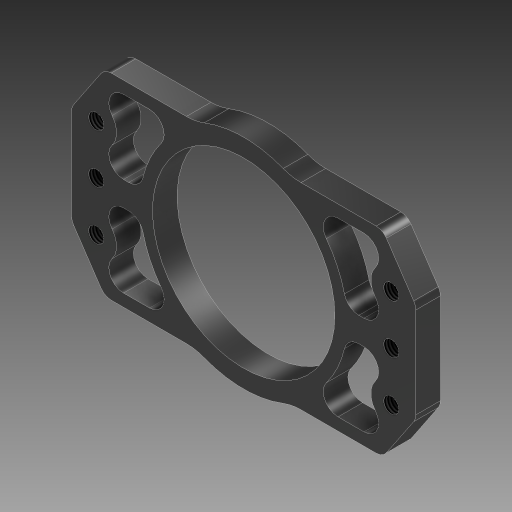
# Autodesk Inventor part: MaxSpline Bearing Block V2
Saved by Autodesk Inventor 2024 (Build 280153000, 153)
## iProperties
Created: 2023-06-08
Part Number: MaxSpline Bearing Block V2
Material: Aluminum 6061
Document SubType Name: Modeling
Designer: Max Boord
Mass: 30.6823 g
Surface Area: 80.6531 cm^2
Volume: 11.3638 cm^3
Density: 2.7 g/cm^3
Appearance: Glossy - Black
Author: Max Boord
Mass: 38.2233 g
Surface Area: 90.3275 cm^2
Volume: 14.1568 cm^3
Mass: 45.745 g
Surface Area: 120.143 cm^2
Volume: 16.9426 cm^3
Autodesk Inventor part; units mm, degrees
ref_plane "YZ Plane" through (0, 0, 0) normal (1, 0, 0) x (0, 1, 0)
ref_plane "XZ Plane" through (0, 0, 0) normal (0, 1, 0) x (-1, 0, 0)
ref_plane "XY Plane" through (0, 0, 0) normal (0, 0, 1) x (1, 0, 0)
sketch "98455A727" plane through (0, 0, 0) normal (0, 0, 1) x (1, 0, 0)
  arc A0 (6.9432, -19.2352) -> (14.6893, -14.3571) centre (-11.4447, 18.5524) ccw
  line L0 (6.9432, -19.2352) -> (8.5729, -23.7501)
  arc A1 (8.5729, -23.7501) -> (-8.5729, -23.7501) centre (0, 0) ccw
  line L1 (-8.5729, -23.7501) -> (-6.9432, -19.2352)
  arc A2 (-14.6893, -14.3571) -> (-6.9432, -19.2352) centre (11.4447, 18.5524) ccw
  arc A3 (-19.2113, -12.7369) -> (-14.6893, -14.3571) centre (-15.9789, -10.8358) ccw
  arc A4 (19.2113, -12.7369) -> (-19.2113, -12.7369) centre (0, -1.4378) ccw
  arc A5 (14.6893, -14.3571) -> (19.2113, -12.7369) centre (15.9789, -10.8358) ccw
  circle A6 centre (11.6445, -18.4904) radius 1.25
  circle A7 centre (-11.6445, -18.4904) radius 1.25
  point P0 (0, 0)
sketch "MaxSpline" plane through (0, 0, 0) normal (0, 0, 1) x (1, 0, 0)
  arc A0 (5.3054, -13.2525) -> (8.8243, -11.2209) centre (0, 0) ccw
  arc A1 (-8.8243, -11.2209) -> (-5.3054, -13.2525) centre (0, 0) ccw
  arc A2 (-14.1297, 2.0316) -> (-14.1297, -2.0316) centre (0, 0) ccw
  arc A3 (-5.3054, 13.2525) -> (-8.8243, 11.2209) centre (0, 0) ccw
  arc A4 (8.8243, 11.2209) -> (5.3054, 13.2525) centre (0, 0) ccw
  arc A5 (-4.7209, 11.79) -> (-2.436, 15.2723) centre (-6.072, 15.1672) ccw
  arc A6 (-2.0329, 15.7443) -> (-2.436, 15.2723) centre (-1.9737, 15.2856) ccw
  arc A7 (2.0329, 15.7443) -> (-2.0329, 15.7443) centre (0, 0) ccw
  arc A8 (2.436, 15.2723) -> (2.0329, 15.7443) centre (1.9737, 15.2856) ccw
  arc A9 (2.436, 15.2723) -> (4.7201, 11.7903) centre (6.072, 15.1672) ccw
  arc A10 (7.8507, 9.9828) -> (4.7201, 11.7903) centre (0, 0) ccw
  arc A11 (7.8507, 9.9828) -> (12.0082, 9.7457) centre (10.0992, 12.8421) ccw
  arc A12 (12.6185, 9.6327) -> (12.0082, 9.7457) centre (12.2509, 9.3521) ccw
  arc A13 (14.6514, 6.1116) -> (12.6185, 9.6327) centre (0, 0) ccw
  arc A14 (14.4442, 5.5265) -> (14.6514, 6.1116) centre (14.2246, 5.9336) ccw
  arc A15 (14.4442, 5.5265) -> (12.5707, 1.8075) centre (16.1712, 2.3251) ccw
  arc A16 (12.5707, -1.8075) -> (12.5707, 1.8075) centre (0, 0) ccw
  arc A17 (12.5707, -1.8075) -> (14.4442, -5.5265) centre (16.1712, -2.3251) ccw
  arc A18 (14.6514, -6.1116) -> (14.4442, -5.5265) centre (14.2246, -5.9336) ccw
  arc A19 (12.6185, -9.6327) -> (14.6514, -6.1116) centre (0, 0) ccw
  arc A20 (12.0082, -9.7457) -> (12.6185, -9.6327) centre (12.2509, -9.3521) ccw
  arc A21 (12.0082, -9.7457) -> (7.8507, -9.9828) centre (10.0992, -12.8421) ccw
  arc A22 (4.7201, -11.7903) -> (7.8507, -9.9828) centre (0, 0) ccw
  arc A23 (4.7201, -11.7903) -> (2.436, -15.2723) centre (6.072, -15.1672) ccw
  arc A24 (2.0329, -15.7443) -> (2.436, -15.2723) centre (1.9737, -15.2856) ccw
  arc A25 (-2.0329, -15.7443) -> (2.0329, -15.7443) centre (0, 0) ccw
  arc A26 (-2.436, -15.2723) -> (-2.0329, -15.7443) centre (-1.9737, -15.2856) ccw
  arc A27 (-2.436, -15.2723) -> (-4.7201, -11.7903) centre (-6.072, -15.1672) ccw
  arc A28 (-7.8507, -9.9828) -> (-4.7201, -11.7903) centre (0, 0) ccw
  arc A29 (-7.8507, -9.9828) -> (-12.0082, -9.7457) centre (-10.0992, -12.8421) ccw
  arc A30 (-12.6185, -9.6327) -> (-12.0082, -9.7457) centre (-12.2509, -9.3521) ccw
  arc A31 (-14.6514, -6.1116) -> (-12.6185, -9.6327) centre (0, 0) ccw
  arc A32 (-14.4442, -5.5265) -> (-14.6514, -6.1116) centre (-14.2246, -5.9336) ccw
  arc A33 (-14.4442, -5.5265) -> (-12.5707, -1.8075) centre (-16.1712, -2.3251) ccw
  arc A34 (-12.5707, 1.8075) -> (-12.5707, -1.8075) centre (0, 0) ccw
  arc A35 (-12.5707, 1.8075) -> (-14.4442, 5.5265) centre (-16.1712, 2.3251) ccw
  arc A36 (-14.6514, 6.1116) -> (-14.4442, 5.5265) centre (-14.2246, 5.9336) ccw
  arc A37 (-12.6185, 9.6327) -> (-14.6514, 6.1116) centre (0, 0) ccw
  arc A38 (-12.0082, 9.7457) -> (-12.6185, 9.6327) centre (-12.2509, 9.3521) ccw
  arc A39 (-12.0082, 9.7457) -> (-7.8507, 9.9828) centre (-10.0992, 12.8421) ccw
  arc A40 (-4.7172, 11.7914) -> (-7.8507, 9.9828) centre (0, 0) ccw
  line L0 (0, 0) -> (0, 22.7025) construction
  line L1 (-1.9737, 15.2856) -> (0, 0) construction
  line L2 (1.9737, 15.2856) -> (0, 0) construction
  line L3 (-10.0992, 12.8421) -> (0, 0) construction
  line L4 (-6.072, 15.1672) -> (0, 0) construction
  arc A41 (2.2346, 17.3063) -> (-2.2346, 17.3063) centre (0, 0) ccw
  arc A42 (16.105, 6.718) -> (13.8704, 10.5884) centre (0, 0) ccw
  arc A43 (13.8704, -10.5884) -> (16.105, -6.718) centre (0, 0) ccw
  arc A44 (-2.2346, -17.3063) -> (2.2346, -17.3063) centre (0, 0) ccw
  arc A45 (-13.8704, 10.5884) -> (-16.105, 6.718) centre (0, 0) ccw
  arc A46 (-16.105, -6.718) -> (-13.8704, -10.5884) centre (0, 0) ccw
  arc A47 (14.1297, -2.0316) -> (14.1297, 2.0316) centre (0, 0) ccw
  dimension "d113" = 360
  dimension "d114" = 2.0375
  dimension "d115" = 2.0625
  dimension "d108" = 14.715
  dimension "d109" = 16.364
  dimension "d110" = 34.9
  dimension "d111" = 28.55
  dimension "d112" = 25.4
  measures "d108" angle of L2 L1
  measures "d109" angle of L3 L4
  measures "d110" diameter of A41
  measures "d111" diameter of A4
  measures "d112" diameter of A10
sketch "Sketch2" plane through (0, 0, 0) normal (0, 0, 1) x (1, 0, 0)
  line L0 (-44.45, 25.4) -> (-44.45, -25.3997)
  circle A0 centre (38.1, 12.7) radius 1.27
  line L1 (44.45, -25.4) -> (-44.45, -25.4)
  line L2 (-44.45, -25.4) -> (-44.45, 25.4)
  line L3 (-44.45, 25.4) -> (44.45, 25.4)
  line L4 (44.45, 25.4) -> (44.45, -25.4)
  line L5 (44.45, -25.4) -> (-44.45, 25.4) construction
  line L6 (-44.45, -25.4) -> (44.45, 25.4) construction
  line L7 (0, 0) -> (0, 25.4) construction
  circle A1 centre (-38.1, -12.7) radius 1.27
  circle A2 centre (-38.1, 12.7) radius 1.27
  circle A3 centre (38.1, -12.7) radius 1.27
  circle A4 centre (0, 0) radius 23.55
  circle A5 centre (0, 0) radius 17.78
  circle A6 centre (0, 0) radius 25 construction
  circle A7 centre (38.1, 12.7) radius 5.2705 construction
  circle A8 centre (-38.1, -12.7) radius 5.2705 construction
  circle A9 centre (-38.1, 12.7) radius 5.2705 construction
  circle A10 centre (38.1, -12.7) radius 5.2705 construction
  line L8 (-44.45, 12.7) -> (-35.9155, 25.4)
  line L9 (44.45, -12.7) -> (35.9155, -25.4)
  line L10 (44.45, 12.7) -> (35.9155, 25.4)
  line L11 (-44.45, -12.7) -> (-35.9155, -25.4)
  circle A11 centre (0, 0) radius 28.175
  circle A12 centre (38.1, 0) radius 1.27
  circle A13 centre (-38.1, 0) radius 1.27
  point P0 (-44.582, -25.3997)
  point P1 (-44.45, 0)
  point P2 (-127, 12.7)
  point P3 (-127, -12.7)
  point P4 (44.45, -12.7)
  point P5 (-44.45, 0)
  dimension "d7" = 2.54
  dimension "d15" = 360
  dimension "d17" = 76.2
  dimension "d18" = 25.4
  dimension "d19" = 47.1
  dimension "d20" = 35.56
  dimension "d21" = 6.35
  dimension "d22" = 50
  dimension "d26" = 360
  dimension "d28" = 10.541
  dimension "d33" = 360
  dimension "d36" = 3.175
  dimension "d37" = 25.4
  dimension "d58" = 50.8
  dimension "d59" = 6.35
  constraints: 22 end point, 14 centre point, 9 symmetric about line, 4 midpoint, 3 coincident, 2 horizontal alignment, 2 parallel, 2 point on line, 1 equal radius, 1 horizontal, 1 perpendicular, 1 tangent, 1 vertical alignment, 24 other
  measures "d7" diameter of A0
  measures "d17" distance of A0.centre A2.centre
  measures "d18" distance of A1.centre A2.centre
  measures "d19" diameter of A4
  measures "d20" diameter of A5
  measures "d22" diameter of A6
  measures "d28" diameter of A7
  measures "d36" radial gap between concentric circles of A6 A11
  measures "d37" distance of L11.start L8.start
  measures "d58" distance between parallel lines of L3 L1
  measures "d59" distance from line of A2.centre L2
extrude "Extrusion3" add sketch "Sketch2" along normal mid plane 6.35 contours L8 L3 A11 L1 L11 L0 | A11 L3 | L3 A11 L1 | L3 L10 L4 L9 L1 A11 | L1 A11
sketch "Sketch3" plane through (0, 0, 3.175) normal (0, 0, 1) x (1, 0, 0)
  point P0 (0, 0)
fillet "Fillet2" radius 3.175 8 edges at (-35.9155, -25.4, 0) (-44.45, -12.7, 0) (-44.45, 12.7, 0) (-35.9155, 25.4, 0) (35.9155, 25.4, 0) (44.45, 12.7, 0) (44.45, -12.7, 0) (35.9155, -25.4, 0)
fillet "Fillet2" radius 12.7 4 edges at (-12.1931, -25.4, 0) (12.1931, -25.4, 0) (12.1931, 25.4, 0) (-12.1931, 25.4, 0)
sketch "Sketch6" plane through (0, 0, 3.175) normal (0, 0, 1) x (1, 0, 0)
  arc A0 (34.2239, -25.4) -> (36.8591, -23.9959) centre (34.2239, -22.225) ccw projected
  line L0 (36.8591, -23.9959) -> (43.9102, -13.5032) projected
  arc A1 (43.9102, -13.5032) -> (44.45, -11.7323) centre (41.275, -11.7323) ccw projected
  line L1 (44.45, -11.7323) -> (44.45, 11.7323) projected
  arc A2 (44.45, 11.7323) -> (43.9102, 13.5032) centre (41.275, 11.7323) ccw projected
  line L2 (43.9102, 13.5032) -> (36.8591, 23.9959) projected
  arc A3 (36.8591, 23.9959) -> (34.2239, 25.4) centre (34.2239, 22.225) ccw projected
  line L3 (34.2239, 25.4) -> (14.8039, 25.4) projected
  arc A4 (10.2043, 26.2622) -> (14.8039, 25.4) centre (14.8039, 38.1) ccw projected
  arc A5 (10.2043, 26.2622) -> (-10.2043, 26.2622) centre (0, 0) ccw projected
  arc A6 (-14.8039, 25.4) -> (-10.2043, 26.2622) centre (-14.8039, 38.1) ccw projected
  line L4 (-14.8039, 25.4) -> (-34.2239, 25.4) projected
  arc A7 (-34.2239, 25.4) -> (-36.8591, 23.9959) centre (-34.2239, 22.225) ccw projected
  line L5 (-36.8591, 23.9959) -> (-43.9102, 13.5032) projected
  arc A8 (-43.9102, 13.5032) -> (-44.45, 11.7323) centre (-41.275, 11.7323) ccw projected
  line L6 (-44.45, 11.7323) -> (-44.45, -11.7323) projected
  arc A9 (-44.45, -11.7323) -> (-43.9102, -13.5032) centre (-41.275, -11.7323) ccw projected
  line L7 (-43.9102, -13.5032) -> (-36.8591, -23.9959) projected
  arc A10 (-36.8591, -23.9959) -> (-34.2239, -25.4) centre (-34.2239, -22.225) ccw projected
  line L8 (-34.2239, -25.4) -> (-14.8039, -25.4) projected
  arc A11 (-10.2043, -26.2622) -> (-14.8039, -25.4) centre (-14.8039, -38.1) ccw projected
  arc A12 (-10.2043, -26.2622) -> (10.2043, -26.2622) centre (0, 0) ccw projected
  arc A13 (14.8039, -25.4) -> (10.2043, -26.2622) centre (14.8039, -38.1) ccw projected
  line L9 (14.8039, -25.4) -> (34.2239, -25.4) projected
  circle A14 centre (0, 0) radius 23.55 projected
  circle A15 centre (38.1, 12.7) radius 1.27 projected
  circle A16 centre (38.1, -12.7) radius 1.27 projected
  circle A17 centre (38.1, 0) radius 1.27 projected
  circle A18 centre (-38.1, -12.7) radius 1.27 projected
  circle A19 centre (-38.1, 12.7) radius 1.27 projected
  circle A20 centre (-38.1, 0) radius 1.27 projected
  circle A21 centre (0, 0) radius 26.725
  line L10 (34.2239, -22.225) -> (41.275, -11.7323)
  line L11 (41.275, -11.7323) -> (41.275, 11.7323)
  line L12 (41.275, 11.7323) -> (34.2239, 22.225)
  line L13 (34.2239, 22.225) -> (14.8039, 22.225)
  arc A22 (9.0544, 23.3028) -> (14.8039, 22.225) centre (14.8039, 38.1) ccw
  arc A23 (9.0544, 23.3028) -> (-9.0544, 23.3028) centre (0, 0) ccw
  arc A24 (-14.8039, 22.225) -> (-9.0544, 23.3028) centre (-14.8039, 38.1) ccw
  line L14 (-14.8039, 22.225) -> (-34.2239, 22.225)
  line L15 (-34.2239, 22.225) -> (-41.275, 11.7323)
  line L16 (-41.275, 11.7323) -> (-41.275, -11.7323)
  line L17 (-41.275, -11.7323) -> (-34.2239, -22.225)
  line L18 (-34.2239, -22.225) -> (-14.8039, -22.225)
  arc A25 (-9.0544, -23.3028) -> (-14.8039, -22.225) centre (-14.8039, -38.1) ccw
  arc A26 (-9.0544, -23.3028) -> (9.0544, -23.3028) centre (0, 0) ccw
  arc A27 (14.8039, -22.225) -> (9.0544, -23.3028) centre (14.8039, -38.1) ccw
  line L19 (14.8039, -22.225) -> (34.2239, -22.225)
  circle A28 centre (38.1, -12.7) radius 5.2705
  circle A29 centre (38.1, 0) radius 5.2705
  circle A30 centre (38.1, 12.7) radius 5.2705
  line L20 (38.1, 0) -> (0, 0) construction
  line L21 (38.1, 3.175) -> (0, 3.175)
  line L22 (0, -3.175) -> (38.1, -3.175)
  arc A31 (38.1, -3.175) -> (38.1, 3.175) centre (38.1, 0) ccw
  arc A32 (0, 3.175) -> (0, -3.175) centre (0, 0) ccw
  line L23 (38.1, -12.7) -> (38.1, 12.7) construction
  line L24 (40.4813, -12.7) -> (40.4813, 12.7)
  line L25 (35.7188, 12.7) -> (35.7188, -12.7)
  arc A33 (35.7188, -12.7) -> (40.4813, -12.7) centre (38.1, -12.7) ccw
  arc A34 (40.4813, 12.7) -> (35.7188, 12.7) centre (38.1, 12.7) ccw
  point P0 (19.05, 0)
  point P1 (38.1, 0)
  point P2 (35.7188, 4.7019)
  point P3 (35.7188, 7.9981)
  point P4 (37.1419, 17.8827)
  point P5 (14.8417, 22.225)
  point P6 (26.5357, 3.175)
  point P7 (33.8932, 3.175)
  point P8 (35.7188, -7.9981)
  point P9 (35.7188, -4.7019)
  point P10 (33.8932, -3.175)
  point P11 (26.5357, -3.175)
  point P12 (14.8417, -22.225)
  point P13 (37.1419, -17.8827)
  dimension "d62" = 3.175
  dimension "d63" = 3.175
  dimension "d64" = 10.541
  dimension "d65" = 6.35
  dimension "d66" = 4.7625
  constraints: 36 end point, 20 point on circle, 14 centre point, 8 tangent, 2 equal radius, 2 midpoint, 2 parallel, 1 horizontal, 1 perpendicular, 15 other
  measures "d62" radial gap between concentric circles of A14 A21
  measures "d63" distance between parallel lines of L9 L19
  measures "d64" diameter of A28
  measures "d65" diameter of A32
  measures "d66" diameter of A34
extrude "Extrusion5" cut sketch "Sketch6" against normal through all contours L10 L19 A21 L22 A29 L25 A28 | L21 A21 L13 L12 A30 L25 A29
fillet "Fillet3" radius 3.81 14 edges at (33.8932, 3.175, 0) (35.7188, 4.7019, 0) (35.7188, 7.9981, 0) (37.1419, 17.8827, 0) (34.2239, 22.225, 0) (14.8417, 22.225, 0) (26.5357, 3.175, 0) (37.1419, -17.8827, 0) (35.7188, -7.9981, 0) (35.7188, -4.7019, 0) (33.8932, -3.175, 0) (26.5357, -3.175, 0) (14.8417, -22.225, 0) (34.2239, -22.225, 0)
mirror "Mirror1" about plane through (0, 0, 0) normal (1, 0, 0) of "Fillet3", "Extrusion5"
sketch "Sketch7" plane through (0, 0, 0) normal (0, 1, 0) x (-1, 0, 0)
  line L0 (21.3614, -3.786) -> (21.3614, 2.325)
  line L1 (21.3614, 2.325) -> (27.7114, 2.325)
  line L2 (27.7114, 2.325) -> (27.7114, 3.214)
  line L3 (5.1562, 3.214) -> (5.1562, -3.786)
  line L4 (0, 0) -> (0, 6.5668)
  line L5 (7.5184, 3.214) -> (7.5184, 2.833)
  line L6 (7.5184, 2.833) -> (18.9992, 2.833)
  line L7 (18.9992, 2.833) -> (18.9992, 3.214)
  line L8 (5.1562, -0.286) -> (21.3614, -0.286) construction
  line L9 (7.5184, -3.786) -> (7.5184, -3.405)
  line L10 (7.5184, -3.405) -> (18.9992, -3.405)
  line L11 (18.9992, -3.405) -> (18.9992, -3.786)
  line L12 (27.7114, 3.214) -> (7.5184, 3.214)
  line L13 (18.9992, 3.214) -> (5.1562, 3.214)
  line L14 (5.1562, -3.786) -> (18.9992, -3.786)
  line L15 (7.5184, -3.786) -> (21.3614, -3.786)
  line L16 (0, 3.175) -> (-3.0494, 3.175) construction
  line L17 (0, 0) -> (-3.6555, 0)
  line L18 (0, -3.175) -> (-3.0494, -3.175) construction
  point P0 (5.1562, 4.675)
  point P1 (13.2588, -3.405)
  point P2 (13.2588, -0.286)
  point P3 (7.5184, -3.786)
  point P4 (18.9992, 3.214)
  point P5 (7.5184, 3.214)
  point P6 (18.9992, -3.786)
  point P7 (18.9992, -3.786)
  point P8 (7.5184, 3.214)
  dimension "d72" = 10.3124
  dimension "d73" = 42.7228
  dimension "d74" = 55.4228
  dimension "d84" = 37.9984
  dimension "d85" = 0.889
  dimension "d87" = 0.381
  dimension "d88" = 7
  dimension "d90" = 6.35
  dimension "d91" = 5.5
  constraints: 38 end point, 8 perpendicular, 6 symmetric about line, 5 horizontal, 3 midpoint, 3 point on line, 2 parallel, 1 collinear, 1 vertical, 1 vertical alignment
  measures "d72" diameter of L3 L4
  measures "d73" diameter of L0 L4
  measures "d74" diameter of L2 L4
  measures "d84" diameter of L7 L4
  measures "d85" distance between parallel lines of L12 L1
  measures "d87" distance between parallel lines of L6 L13
  measures "d88" distance of L3.start L3.end
  measures "d90" distance between parallel lines of L18 L16
  measures "d91" distance between parallel lines of L1 L18
revolve "Revolution1" [suppressed]
delete_face "Delete Face1" [suppressed]
ref_plane "Work Plane3" through (0, 0, 3.2258) normal (0, 0, 1) x (1, 0, 0)
sketch "Sketch8" plane through (0, 0, 3.2258) normal (0, 0, 1) x (1, 0, 0)
  circle A0 centre (0, 0) radius 24.75
  dimension "d92" = 49.5
  constraints: 1 centre point, 1 coincident
  measures "d92" diameter of A0
extrude "Extrusion6" [suppressed]
sketch "Sketch9" plane through (0, 0, -3.175) normal (0, 0, -1) x (-1, 0, 0)
  circle A0 centre (0, 0) radius 23.55 projected
  circle A1 centre (0, 0) radius 19.0119
  dimension "d95" = 38.0238
  constraints: 1 centre point
  measures "d95" diameter of A1
extrude "Extrusion7" [suppressed]
sketch "Sketch10" plane through (0, 0, 3.175) normal (0, 0, 1) x (1, 0, 0)
  arc A0 (6.9432, -19.2352) -> (14.6893, -14.3571) centre (-11.4447, 18.5524) ccw
  line L0 (6.9432, -19.2352) -> (8.5729, -23.7501)
  arc A1 (8.5729, -23.7501) -> (-8.5729, -23.7501) centre (0, 0) ccw
  line L1 (-8.5729, -23.7501) -> (-6.9432, -19.2352)
  arc A2 (-14.6893, -14.3571) -> (-6.9432, -19.2352) centre (11.4447, 18.5524) ccw
  arc A3 (-19.2113, -12.7369) -> (-14.6893, -14.3571) centre (-15.9789, -10.8358) ccw
  arc A4 (19.2113, -12.7369) -> (-19.2113, -12.7369) centre (0, -1.4378) ccw
  arc A5 (14.6893, -14.3571) -> (19.2113, -12.7369) centre (15.9789, -10.8358) ccw
  circle A6 centre (11.6445, -18.4904) radius 1.25
  circle A7 centre (-11.6445, -18.4904) radius 1.25
  point P0 (0, 0)
  constraints: 1 other
extrude "Extrusion8" [suppressed]
sketch "Sketch11" plane through (0, 0, 3.175) normal (0, 0, 1) x (1, 0, 0)
  circle A0 centre (-38.1, 12.7) radius 1.27 projected
  circle A1 centre (-38.1, 0) radius 1.27 projected
  circle A2 centre (-38.1, -12.7) radius 1.27 projected
  circle A3 centre (38.1, 12.7) radius 1.27 projected
  circle A4 centre (38.1, 0) radius 1.27 projected
  circle A5 centre (38.1, -12.7) radius 1.27 projected
  point P0 (0, 0)
  constraints: 6 coincident
hole "Hole1" at (-38.1, 12.7, 3.175) at (-38.1, 0, 3.175) at (-38.1, -12.7, 3.175) at (38.1, 12.7, 3.175) at (38.1, 0, 3.175) at (38.1, -12.7, 3.175) direction (0, 0, -1) diameter 3.9624 end through all thread size "10-32 UNF" class "2B" standard "ANSI Unified Screw Threads"
sketch "Sketch12" plane through (0, 0, 3.175) normal (0, 0, 1) x (1, 0, 0)
  circle A0 centre (0, 0) radius 23.55 projected
  arc A1 (10.5884, 13.8704) -> (6.718, 16.105) centre (0, 0) ccw
  arc A2 (6.718, 16.105) -> (4.1403, 15.1919) centre (5.9336, 14.2246) ccw
  arc A3 (2.0316, 14.1297) -> (4.1403, 15.1919) centre (2.3251, 16.1712) ccw
  arc A4 (2.0316, 14.1297) -> (-2.0316, 14.1297) centre (0, 0) ccw
  arc A5 (-4.1403, 15.1919) -> (-2.0316, 14.1297) centre (-2.3251, 16.1712) ccw
  arc A6 (-4.1403, 15.1919) -> (-6.718, 16.105) centre (-5.9336, 14.2246) ccw
  arc A7 (-6.718, 16.105) -> (-10.5884, 13.8704) centre (0, 0) ccw
  arc A8 (-10.5884, 13.8704) -> (-11.0864, 11.1816) centre (-9.3521, 12.2509) ccw
  arc A9 (-11.2209, 8.8243) -> (-11.0864, 11.1816) centre (-12.8421, 10.0992) ccw
  arc A10 (-11.2209, 8.8243) -> (-13.2525, 5.3054) centre (0, 0) ccw
  arc A11 (-15.2268, 4.0103) -> (-13.2525, 5.3054) centre (-15.1672, 6.072) ccw
  arc A12 (-15.2268, 4.0103) -> (-17.3063, 2.2346) centre (-15.2856, 1.9737) ccw
  arc A13 (-17.3063, 2.2346) -> (-17.3063, -2.2346) centre (0, 0) ccw
  arc A14 (-17.3063, -2.2346) -> (-15.2268, -4.0103) centre (-15.2856, -1.9737) ccw
  arc A15 (-13.2525, -5.3054) -> (-15.2268, -4.0103) centre (-15.1672, -6.072) ccw
  arc A16 (-13.2525, -5.3054) -> (-11.2209, -8.8243) centre (0, 0) ccw
  arc A17 (-11.0864, -11.1816) -> (-11.2209, -8.8243) centre (-12.8421, -10.0992) ccw
  arc A18 (-11.0864, -11.1816) -> (-10.5884, -13.8704) centre (-9.3521, -12.2509) ccw
  arc A19 (-10.5884, -13.8704) -> (-6.718, -16.105) centre (0, 0) ccw
  arc A20 (-6.718, -16.105) -> (-4.1403, -15.1919) centre (-5.9336, -14.2246) ccw
  arc A21 (-2.0316, -14.1297) -> (-4.1403, -15.1919) centre (-2.3251, -16.1712) ccw
  arc A22 (-2.0316, -14.1297) -> (2.0316, -14.1297) centre (0, 0) ccw
  arc A23 (4.1403, -15.1919) -> (2.0316, -14.1297) centre (2.3251, -16.1712) ccw
  arc A24 (4.1403, -15.1919) -> (6.718, -16.105) centre (5.9336, -14.2246) ccw
  arc A25 (6.718, -16.105) -> (10.5884, -13.8704) centre (0, 0) ccw
  arc A26 (10.5884, -13.8704) -> (11.0864, -11.1816) centre (9.3521, -12.2509) ccw
  arc A27 (11.2209, -8.8243) -> (11.0864, -11.1816) centre (12.8421, -10.0992) ccw
  arc A28 (11.2209, -8.8243) -> (13.2525, -5.3054) centre (0, 0) ccw
  arc A29 (15.2268, -4.0103) -> (13.2525, -5.3054) centre (15.1672, -6.072) ccw
  arc A30 (15.2268, -4.0103) -> (17.3063, -2.2346) centre (15.2856, -1.9737) ccw
  arc A31 (17.3063, -2.2346) -> (17.3063, 2.2346) centre (0, 0) ccw
  arc A32 (17.3063, 2.2346) -> (15.2268, 4.0103) centre (15.2856, 1.9737) ccw
  arc A33 (13.2525, 5.3054) -> (15.2268, 4.0103) centre (15.1672, 6.072) ccw
  arc A34 (13.2525, 5.3054) -> (11.2209, 8.8243) centre (0, 0) ccw
  arc A35 (11.0864, 11.1816) -> (11.2209, 8.8243) centre (12.8421, 10.0992) ccw
  arc A36 (11.0864, 11.1816) -> (10.5884, 13.8704) centre (9.3521, 12.2509) ccw
  arc A37 (6.1116, 14.6514) -> (5.5265, 14.4442) centre (5.9336, 14.2246) ccw
  arc A38 (9.6327, 12.6185) -> (6.1116, 14.6514) centre (0, 0) ccw
  arc A39 (9.7457, 12.0082) -> (9.6327, 12.6185) centre (9.3521, 12.2509) ccw
  arc A40 (9.7457, 12.0082) -> (9.9828, 7.8507) centre (12.8421, 10.0992) ccw
  arc A41 (11.7903, 4.7201) -> (9.9828, 7.8507) centre (0, 0) ccw
  arc A42 (11.7903, 4.7201) -> (15.2723, 2.436) centre (15.1672, 6.072) ccw
  arc A43 (15.7443, 2.0329) -> (15.2723, 2.436) centre (15.2856, 1.9737) ccw
  arc A44 (15.7443, -2.0329) -> (15.7443, 2.0329) centre (0, 0) ccw
  arc A45 (15.2723, -2.436) -> (15.7443, -2.0329) centre (15.2856, -1.9737) ccw
  arc A46 (15.2723, -2.436) -> (11.7903, -4.7201) centre (15.1672, -6.072) ccw
  arc A47 (9.9828, -7.8507) -> (11.7903, -4.7201) centre (0, 0) ccw
  arc A48 (9.9828, -7.8507) -> (9.7457, -12.0082) centre (12.8421, -10.0992) ccw
  arc A49 (9.6327, -12.6185) -> (9.7457, -12.0082) centre (9.3521, -12.2509) ccw
  arc A50 (6.1116, -14.6514) -> (9.6327, -12.6185) centre (0, 0) ccw
  arc A51 (5.5265, -14.4442) -> (6.1116, -14.6514) centre (5.9336, -14.2246) ccw
  arc A52 (5.5265, -14.4442) -> (1.8075, -12.5707) centre (2.3251, -16.1712) ccw
  arc A53 (-1.8075, -12.5707) -> (1.8075, -12.5707) centre (0, 0) ccw
  arc A54 (-1.8075, -12.5707) -> (-5.5265, -14.4442) centre (-2.3251, -16.1712) ccw
  arc A55 (-6.1116, -14.6514) -> (-5.5265, -14.4442) centre (-5.9336, -14.2246) ccw
  arc A56 (-9.6327, -12.6185) -> (-6.1116, -14.6514) centre (0, 0) ccw
  arc A57 (-9.7457, -12.0082) -> (-9.6327, -12.6185) centre (-9.3521, -12.2509) ccw
  arc A58 (-9.7457, -12.0082) -> (-9.9828, -7.8507) centre (-12.8421, -10.0992) ccw
  arc A59 (-11.7903, -4.7201) -> (-9.9828, -7.8507) centre (0, 0) ccw
  arc A60 (-11.7903, -4.7201) -> (-15.2723, -2.436) centre (-15.1672, -6.072) ccw
  arc A61 (-15.7443, -2.0329) -> (-15.2723, -2.436) centre (-15.2856, -1.9737) ccw
  arc A62 (-15.7443, 2.0329) -> (-15.7443, -2.0329) centre (0, 0) ccw
  arc A63 (-15.2723, 2.436) -> (-15.7443, 2.0329) centre (-15.2856, 1.9737) ccw
  arc A64 (-15.2723, 2.436) -> (-11.7903, 4.7201) centre (-15.1672, 6.072) ccw
  arc A65 (-9.9828, 7.8507) -> (-11.7903, 4.7201) centre (0, 0) ccw
  arc A66 (-9.9828, 7.8507) -> (-9.7457, 12.0082) centre (-12.8421, 10.0992) ccw
  arc A67 (-9.6327, 12.6185) -> (-9.7457, 12.0082) centre (-9.3521, 12.2509) ccw
  arc A68 (-6.1116, 14.6514) -> (-9.6327, 12.6185) centre (0, 0) ccw
  arc A69 (-5.5265, 14.4442) -> (-6.1116, 14.6514) centre (-5.9336, 14.2246) ccw
  arc A70 (-5.5265, 14.4442) -> (-1.8075, 12.5707) centre (-2.3251, 16.1712) ccw
  arc A71 (1.8066, 12.5708) -> (-1.8075, 12.5707) centre (0, 0) ccw
  arc A72 (1.8066, 12.5708) -> (5.5265, 14.4442) centre (2.3251, 16.1712) ccw
  constraints: 1 other
extrude "Extrusion9" [suppressed]
thicken "Thicken1" [suppressed]
delete_face "Delete Face2" [suppressed]
sketch "Sketch13" plane through (-34.2239, -25.4, 3.175) normal (0, 0, 1) x (1, 0, 0)
  line L0 (58.5811, 47.625) -> (65.2674, 47.625) projected
  arc A0 (68.2281, 41.4171) -> (65.2674, 47.625) centre (65.2674, 43.815) ccw projected
  arc A1 (68.2281, 41.4171) -> (68.2281, 34.7829) centre (72.3239, 38.1) ccw projected
  arc A2 (65.2674, 28.575) -> (68.2281, 34.7829) centre (65.2674, 32.385) ccw projected
  line L1 (65.2674, 28.575) -> (63.9492, 28.575) projected
  arc A3 (60.2402, 31.5134) -> (63.9492, 28.575) centre (63.9492, 32.385) ccw projected
  arc A4 (60.2402, 31.5134) -> (55.5419, 41.5173) centre (34.2239, 25.4) ccw projected
  arc A5 (58.5811, 47.625) -> (55.5419, 41.5173) centre (58.5811, 43.815) ccw projected
  line L2 (0, 0) -> (19.42, 0) projected
  arc A6 (68.4477, 0) -> (71.083, 1.4041) centre (68.4477, 3.175) ccw projected
  line L3 (71.083, 1.4041) -> (78.1341, 11.8968) projected
  arc A7 (78.1341, 11.8968) -> (78.6739, 13.6677) centre (75.4989, 13.6677) ccw projected
  line L4 (78.6739, 13.6677) -> (78.6739, 37.1323) projected
  arc A8 (78.6739, 37.1323) -> (78.1341, 38.9032) centre (75.4989, 37.1323) ccw projected
  line L5 (78.1341, 38.9032) -> (71.083, 49.3959) projected
  arc A9 (71.083, 49.3959) -> (68.4477, 50.8) centre (68.4477, 47.625) ccw projected
  line L6 (68.4477, 50.8) -> (49.0278, 50.8) projected
  arc A10 (0, 50.8) -> (-2.6352, 49.3959) centre (0, 47.625) ccw projected
  line L7 (-2.6352, 49.3959) -> (-9.6864, 38.9032) projected
  arc A11 (-9.6864, 38.9032) -> (-10.2261, 37.1323) centre (-7.0511, 37.1323) ccw projected
  line L8 (-10.2261, 37.1323) -> (-10.2261, 13.6677) projected
  arc A12 (-10.2261, 13.6677) -> (-9.6864, 11.8968) centre (-7.0511, 13.6677) ccw projected
  line L9 (-9.6864, 11.8968) -> (-2.6352, 1.4041) projected
  arc A13 (-2.6352, 1.4041) -> (0, 0) centre (0, 3.175) ccw projected
  circle A14 centre (72.3239, 12.7) radius 1.9812 projected
  circle A15 centre (72.3239, 25.4) radius 1.9812 projected
  circle A16 centre (72.3239, 38.1) radius 1.9812 projected
  circle A17 centre (-3.8761, 12.7) radius 1.9812 projected
  circle A18 centre (-3.8761, 25.4) radius 1.9812 projected
  circle A19 centre (-3.8761, 38.1) radius 1.9812 projected
  line L10 (3.1804, 22.225) -> (4.4985, 22.225) projected
  arc A20 (8.2075, 19.2866) -> (4.4985, 22.225) centre (4.4985, 18.415) ccw projected
  arc A21 (8.2075, 19.2866) -> (12.9058, 9.2827) centre (34.2239, 25.4) ccw projected
  arc A22 (9.8666, 3.175) -> (12.9058, 9.2827) centre (9.8666, 6.985) ccw projected
  line L11 (9.8666, 3.175) -> (3.1804, 3.175) projected
  arc A23 (0.2196, 9.3829) -> (3.1804, 3.175) centre (3.1804, 6.985) ccw projected
  arc A24 (0.2196, 9.3829) -> (0.2196, 16.0171) centre (-3.8761, 12.7) ccw projected
  arc A25 (3.1804, 22.225) -> (0.2196, 16.0171) centre (3.1804, 18.415) ccw projected
  line L12 (3.1804, 47.625) -> (9.8666, 47.625) projected
  arc A26 (12.9058, 41.5173) -> (9.8666, 47.625) centre (9.8666, 43.815) ccw projected
  arc A27 (12.9058, 41.5173) -> (8.2075, 31.5134) centre (34.2239, 25.4) ccw projected
  arc A28 (4.4985, 28.575) -> (8.2075, 31.5134) centre (4.4985, 32.385) ccw projected
  line L13 (4.4985, 28.575) -> (3.1804, 28.575) projected
  arc A29 (0.2196, 34.7829) -> (3.1804, 28.575) centre (3.1804, 32.385) ccw projected
  arc A30 (0.2196, 34.7829) -> (0.2196, 41.4171) centre (-3.8761, 38.1) ccw projected
  arc A31 (3.1804, 47.625) -> (0.2196, 41.4171) centre (3.1804, 43.815) ccw projected
  arc A32 (68.2281, 16.0171) -> (68.2281, 9.3829) centre (72.3239, 12.7) ccw projected
  arc A33 (65.2674, 3.175) -> (68.2281, 9.3829) centre (65.2674, 6.985) ccw projected
  line L14 (65.2674, 3.175) -> (58.5811, 3.175) projected
  arc A34 (55.5419, 9.2827) -> (58.5811, 3.175) centre (58.5811, 6.985) ccw projected
  arc A35 (55.5419, 9.2827) -> (60.2402, 19.2866) centre (34.2239, 25.4) ccw projected
  arc A36 (63.9492, 22.225) -> (60.2402, 19.2866) centre (63.9492, 18.415) ccw projected
  line L15 (63.9492, 22.225) -> (65.2674, 22.225) projected
  arc A37 (68.2281, 16.0171) -> (65.2674, 22.225) centre (65.2674, 18.415) ccw projected
  arc A38 (50.3039, 47.625) -> (47.7979, 40.9451) centre (50.3039, 43.815) ccw
  line L16 (50.3039, 47.625) -> (58.5811, 47.625)
  arc A39 (58.5811, 47.625) -> (55.5419, 41.5173) centre (58.5811, 43.815) ccw projected
  line L17 (63.9492, 28.575) -> (57.6523, 28.575)
  arc A40 (54.0011, 31.2964) -> (57.6523, 28.575) centre (57.6523, 32.385) ccw
  arc A41 (60.2402, 31.5134) -> (63.9492, 28.575) centre (63.9492, 32.385) ccw projected
  arc A42 (54.0011, 31.2964) -> (47.7979, 40.9451) centre (34.2239, 25.4) ccw
  arc A43 (44.8729, 39.3499) -> (40.9803, 41.5973) centre (34.2239, 25.4) ccw projected
  line L18 (34.2239, 25.4) -> (34.2239, 31.4123)
  line L19 (34.2239, 25.4) -> (40.9803, 25.4)
  arc A44 (20.6498, 40.9451) -> (18.1438, 47.625) centre (18.1438, 43.815) ccw
  line L20 (18.1438, 47.625) -> (9.8666, 47.625)
  line L21 (4.4985, 28.575) -> (10.7955, 28.575)
  arc A45 (10.7955, 28.575) -> (14.4466, 31.2964) centre (10.7955, 32.385) ccw
  arc A46 (20.6498, 40.9451) -> (14.4466, 31.2964) centre (34.2239, 25.4) ccw
  arc A47 (47.7979, 9.8549) -> (50.3039, 3.175) centre (50.3039, 6.985) ccw
  line L22 (50.3039, 3.175) -> (58.5811, 3.175)
  line L23 (63.9492, 22.225) -> (57.6523, 22.225)
  arc A48 (57.6523, 22.225) -> (54.0011, 19.5036) centre (57.6523, 18.415) ccw
  arc A49 (47.7979, 9.8549) -> (54.0011, 19.5036) centre (34.2239, 25.4) ccw
  arc A50 (18.1438, 3.175) -> (20.6498, 9.8549) centre (18.1438, 6.985) ccw
  arc A51 (14.4466, 19.5036) -> (20.6498, 9.8549) centre (34.2239, 25.4) ccw
  arc A52 (14.4466, 19.5036) -> (10.7955, 22.225) centre (10.7955, 18.415) ccw
  line L24 (4.4985, 22.225) -> (10.7955, 22.225)
  line L25 (18.1438, 3.175) -> (9.8666, 3.175)
  arc A53 (44.4281, 51.6622) -> (49.0278, 50.8) centre (49.0278, 63.5) ccw projected
  arc A54 (44.4281, 51.6622) -> (24.0196, 51.6622) centre (34.2239, 25.4) ccw projected
  arc A55 (19.42, 50.8) -> (24.0196, 51.6622) centre (19.42, 63.5) ccw projected
  line L26 (19.42, 50.8) -> (0, 50.8) projected
  arc A56 (24.0196, -0.8622) -> (19.42, 0) centre (19.42, -12.7) ccw projected
  arc A57 (24.0196, -0.8622) -> (44.4281, -0.8622) centre (34.2239, 25.4) ccw projected
  arc A58 (49.0278, 0) -> (44.4281, -0.8622) centre (49.0278, -12.7) ccw projected
  line L27 (49.0278, 0) -> (68.4477, 0) projected
  point P0 (9.8666, 3.175)
  point P1 (4.4999, 22.225)
  point P2 (4.4985, 28.575)
  dimension "d130" = 41.275
  constraints: 24 point on circle, 22 symmetric about line, 20 end point, 12 centre point, 5 tangent, 2 equal radius, 2 horizontal, 1 concentric, 1 vertical, 9 other
  measures "d130" diameter of A42
extrude "Extrusion10" [suppressed]
sketch "Block3" plane through (0, 0, 0) normal (0, 0, 1) x (1, 0, 0)
  arc A0 (2.2346, 17.3063) -> (-2.2346, 17.3063) centre (0, 0) ccw
  arc A1 (-2.2346, 17.3063) -> (-4.0103, 15.2268) centre (-1.9737, 15.2856) ccw
  arc A2 (-5.3054, 13.2525) -> (-4.0103, 15.2268) centre (-6.072, 15.1672) ccw
  arc A3 (-5.3054, 13.2525) -> (-8.8243, 11.2209) centre (0, 0) ccw
  arc A4 (-11.1816, 11.0864) -> (-8.8243, 11.2209) centre (-10.0992, 12.8421) ccw
  arc A5 (-11.1816, 11.0864) -> (-13.8704, 10.5884) centre (-12.2509, 9.3521) ccw
  arc A6 (-13.8704, 10.5884) -> (-16.105, 6.718) centre (0, 0) ccw
  arc A7 (-16.105, 6.718) -> (-15.1919, 4.1403) centre (-14.2246, 5.9336) ccw
  arc A8 (-14.1297, 2.0316) -> (-15.1919, 4.1403) centre (-16.1712, 2.3251) ccw
  arc A9 (-14.1297, 2.0316) -> (-14.1297, -2.0316) centre (0, 0) ccw
  arc A10 (-15.1919, -4.1403) -> (-14.1297, -2.0316) centre (-16.1712, -2.3251) ccw
  arc A11 (-15.1919, -4.1403) -> (-16.105, -6.718) centre (-14.2246, -5.9336) ccw
  arc A12 (-16.105, -6.718) -> (-13.8704, -10.5884) centre (0, 0) ccw
  arc A13 (-13.8704, -10.5884) -> (-11.1816, -11.0864) centre (-12.2509, -9.3521) ccw
  arc A14 (-8.8243, -11.2209) -> (-11.1816, -11.0864) centre (-10.0992, -12.8421) ccw
  arc A15 (-8.8243, -11.2209) -> (-5.3054, -13.2525) centre (0, 0) ccw
  arc A16 (-4.0103, -15.2268) -> (-5.3054, -13.2525) centre (-6.072, -15.1672) ccw
  arc A17 (-4.0103, -15.2268) -> (-2.2346, -17.3063) centre (-1.9737, -15.2856) ccw
  arc A18 (-2.2346, -17.3063) -> (2.2346, -17.3063) centre (0, 0) ccw
  arc A19 (2.2346, -17.3063) -> (4.0103, -15.2268) centre (1.9737, -15.2856) ccw
  arc A20 (5.3054, -13.2525) -> (4.0103, -15.2268) centre (6.072, -15.1672) ccw
  arc A21 (5.3054, -13.2525) -> (8.8243, -11.2209) centre (0, 0) ccw
  arc A22 (11.1816, -11.0864) -> (8.8243, -11.2209) centre (10.0992, -12.8421) ccw
  arc A23 (11.1816, -11.0864) -> (13.8704, -10.5884) centre (12.2509, -9.3521) ccw
  arc A24 (13.8704, -10.5884) -> (16.105, -6.718) centre (0, 0) ccw
  arc A25 (16.105, -6.718) -> (15.1919, -4.1403) centre (14.2246, -5.9336) ccw
  arc A26 (14.1297, -2.0316) -> (15.1919, -4.1403) centre (16.1712, -2.3251) ccw
  arc A27 (14.1297, -2.0316) -> (14.1297, 2.0316) centre (0, 0) ccw
  arc A28 (15.1919, 4.1403) -> (14.1297, 2.0316) centre (16.1712, 2.3251) ccw
  arc A29 (15.1919, 4.1403) -> (16.105, 6.718) centre (14.2246, 5.9336) ccw
  arc A30 (16.105, 6.718) -> (13.8704, 10.5884) centre (0, 0) ccw
  arc A31 (13.8704, 10.5884) -> (11.1816, 11.0864) centre (12.2509, 9.3521) ccw
  arc A32 (8.8243, 11.2209) -> (11.1816, 11.0864) centre (10.0992, 12.8421) ccw
  arc A33 (8.8243, 11.2209) -> (5.3054, 13.2525) centre (0, 0) ccw
  arc A34 (4.0103, 15.2268) -> (5.3054, 13.2525) centre (6.072, 15.1672) ccw
  arc A35 (4.0103, 15.2268) -> (2.2346, 17.3063) centre (1.9737, 15.2856) ccw
  arc A36 (-2.0329, 15.7443) -> (-2.436, 15.2723) centre (-1.9737, 15.2856) ccw
  arc A37 (2.0329, 15.7443) -> (-2.0329, 15.7443) centre (0, 0) ccw
  arc A38 (2.436, 15.2723) -> (2.0329, 15.7443) centre (1.9737, 15.2856) ccw
  arc A39 (2.436, 15.2723) -> (4.7201, 11.7903) centre (6.072, 15.1672) ccw
  arc A40 (7.8507, 9.9828) -> (4.7201, 11.7903) centre (0, 0) ccw
  arc A41 (7.8507, 9.9828) -> (12.0082, 9.7457) centre (10.0992, 12.8421) ccw
  arc A42 (12.6185, 9.6327) -> (12.0082, 9.7457) centre (12.2509, 9.3521) ccw
  arc A43 (14.6514, 6.1116) -> (12.6185, 9.6327) centre (0, 0) ccw
  arc A44 (14.4442, 5.5265) -> (14.6514, 6.1116) centre (14.2246, 5.9336) ccw
  arc A45 (14.4442, 5.5265) -> (12.5707, 1.8075) centre (16.1712, 2.3251) ccw
  arc A46 (12.5707, -1.8075) -> (12.5707, 1.8075) centre (0, 0) ccw
  arc A47 (12.5707, -1.8075) -> (14.4442, -5.5265) centre (16.1712, -2.3251) ccw
  arc A48 (14.6514, -6.1116) -> (14.4442, -5.5265) centre (14.2246, -5.9336) ccw
  arc A49 (12.6185, -9.6327) -> (14.6514, -6.1116) centre (0, 0) ccw
  arc A50 (12.0082, -9.7457) -> (12.6185, -9.6327) centre (12.2509, -9.3521) ccw
  arc A51 (12.0082, -9.7457) -> (7.8507, -9.9828) centre (10.0992, -12.8421) ccw
  arc A52 (4.7201, -11.7903) -> (7.8507, -9.9828) centre (0, 0) ccw
  arc A53 (4.7201, -11.7903) -> (2.436, -15.2723) centre (6.072, -15.1672) ccw
  arc A54 (2.0329, -15.7443) -> (2.436, -15.2723) centre (1.9737, -15.2856) ccw
  arc A55 (-2.0329, -15.7443) -> (2.0329, -15.7443) centre (0, 0) ccw
  arc A56 (-2.436, -15.2723) -> (-2.0329, -15.7443) centre (-1.9737, -15.2856) ccw
  arc A57 (-2.436, -15.2723) -> (-4.7201, -11.7903) centre (-6.072, -15.1672) ccw
  arc A58 (-7.8507, -9.9828) -> (-4.7201, -11.7903) centre (0, 0) ccw
  arc A59 (-7.8507, -9.9828) -> (-12.0082, -9.7457) centre (-10.0992, -12.8421) ccw
  arc A60 (-12.6185, -9.6327) -> (-12.0082, -9.7457) centre (-12.2509, -9.3521) ccw
  arc A61 (-14.6514, -6.1116) -> (-12.6185, -9.6327) centre (0, 0) ccw
  arc A62 (-14.4442, -5.5265) -> (-14.6514, -6.1116) centre (-14.2246, -5.9336) ccw
  arc A63 (-14.4442, -5.5265) -> (-12.5707, -1.8075) centre (-16.1712, -2.3251) ccw
  arc A64 (-12.5707, 1.8075) -> (-12.5707, -1.8075) centre (0, 0) ccw
  arc A65 (-12.5707, 1.8075) -> (-14.4442, 5.5265) centre (-16.1712, 2.3251) ccw
  arc A66 (-14.6514, 6.1116) -> (-14.4442, 5.5265) centre (-14.2246, 5.9336) ccw
  arc A67 (-12.6185, 9.6327) -> (-14.6514, 6.1116) centre (0, 0) ccw
  arc A68 (-12.0082, 9.7457) -> (-12.6185, 9.6327) centre (-12.2509, 9.3521) ccw
  arc A69 (-12.0082, 9.7457) -> (-7.8507, 9.9828) centre (-10.0992, 12.8421) ccw
  arc A70 (-4.7209, 11.79) -> (-7.8507, 9.9828) centre (0, 0) ccw
  arc A71 (-4.7209, 11.79) -> (-2.436, 15.2723) centre (-6.072, 15.1672) ccw
  constraints: 144 point on circle, 143 centre point, 1 coincident
body "Solid1"
body "Solid2"
body "Solid3"
